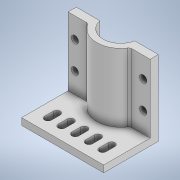
# Autodesk Inventor part: CLAMP
Saved by Autodesk Inventor 2022 (Build 260153000, 153)
## iProperties
Created: 2022-02-10
Part Number: CLAMP
Material: Generic
Document SubType Name: Modeling
Designer: 24sa01
Density: 1 g/cm^3
Appearance: Default
Author: 24sa01
Autodesk Inventor part; units mm, degrees
ref_plane "YZ Plane" through (0, 0, 0) normal (1, 0, 0) x (0, 1, 0)
ref_plane "XZ Plane" through (0, 0, 0) normal (0, 1, 0) x (-1, 0, 0)
ref_plane "XY Plane" through (0, 0, 0) normal (0, 0, 1) x (1, 0, 0)
sketch "Sketch1" plane through (0, 0, 0) normal (0, 1, 0) x (-1, 0, 0)
  line L0 (0, 0) -> (-76.2, 0)
  line L1 (-76.2, 0) -> (-76.2, -50.8)
  line L2 (-76.2, -50.8) -> (0, -50.8)
  line L3 (0, -50.8) -> (0, 0)
  line L4 (-12.7, -11.7475) -> (-12.7, -20.0025) construction
  line L5 (-15.875, -11.7475) -> (-15.875, -20.0025)
  line L6 (-9.525, -20.0025) -> (-9.525, -11.7475)
  arc A0 (-9.525, -11.7475) -> (-15.875, -11.7475) centre (-12.7, -11.7475) ccw
  arc A1 (-15.875, -20.0025) -> (-9.525, -20.0025) centre (-12.7, -20.0025) ccw
  line L7 (-25.4, -11.7475) -> (-25.4, -20.0025) construction
  line L8 (-28.575, -11.7475) -> (-28.575, -20.0025)
  line L9 (-22.225, -20.0025) -> (-22.225, -11.7475)
  arc A2 (-22.225, -11.7475) -> (-28.575, -11.7475) centre (-25.4, -11.7475) ccw
  arc A3 (-28.575, -20.0025) -> (-22.225, -20.0025) centre (-25.4, -20.0025) ccw
  line L10 (-28.575, -11.7475) -> (-28.575, -20.0025)
  line L11 (-25.4, -11.7475) -> (-25.4, -20.0025) construction
  arc A4 (-22.225, -11.7475) -> (-28.575, -11.7475) centre (-25.4, -11.7475) ccw
  line L12 (-22.225, -20.0025) -> (-22.225, -11.7475)
  arc A5 (-28.575, -20.0025) -> (-22.225, -20.0025) centre (-25.4, -20.0025) ccw
  line L13 (-41.275, -11.7475) -> (-41.275, -20.0025)
  line L14 (-38.1, -11.7475) -> (-38.1, -20.0025) construction
  arc A6 (-34.925, -11.7475) -> (-41.275, -11.7475) centre (-38.1, -11.7475) ccw
  line L15 (-34.925, -20.0025) -> (-34.925, -11.7475)
  arc A7 (-41.275, -20.0025) -> (-34.925, -20.0025) centre (-38.1, -20.0025) ccw
  line L16 (-53.975, -11.7475) -> (-53.975, -20.0025)
  line L17 (-50.8, -11.7475) -> (-50.8, -20.0025) construction
  arc A8 (-47.625, -11.7475) -> (-53.975, -11.7475) centre (-50.8, -11.7475) ccw
  line L18 (-47.625, -20.0025) -> (-47.625, -11.7475)
  arc A9 (-53.975, -20.0025) -> (-47.625, -20.0025) centre (-50.8, -20.0025) ccw
  line L19 (-66.675, -11.7475) -> (-66.675, -20.0025)
  line L20 (-63.5, -11.7475) -> (-63.5, -20.0025) construction
  arc A10 (-60.325, -11.7475) -> (-66.675, -11.7475) centre (-63.5, -11.7475) ccw
  line L21 (-60.325, -20.0025) -> (-60.325, -11.7475)
  arc A11 (-66.675, -20.0025) -> (-60.325, -20.0025) centre (-63.5, -20.0025) ccw
  point P0 (-12.7, -15.875)
  point P1 (-25.4, -15.875)
  point P2 (-25.4, -15.875)
  point P3 (-38.1, -15.875)
  point P4 (-50.8, -15.875)
  point P5 (-63.5, -15.875)
  dimension "d0" = 50.8
  dimension "d1" = 76.2
  dimension "d41" = 8.255
  dimension "d42" = 6.35
  dimension "d43" = 12.7
  dimension "d44" = 8.255
  dimension "d45" = 6.35
  dimension "d56" = 12.7
  dimension "d57" = 15.875
  dimension "d60" = 12.7
  constraints: 56 end point, 24 point on circle, 12 centre point, 8 tangent, 4 parallel, 2 horizontal, 2 midpoint, 2 vertical, 1 horizontal alignment, 1 perpendicular, 48 other
  measures "d0" distance of L0.end L1.end
  measures "d1" distance of L1.end L2.end
  measures "d41" distance of L4.start L4.end
  measures "d42" diameter of A1
  measures "d43" distance from line of L3 point (-12.7, -15.875)
  measures "d44" distance of L7.start L7.end
  measures "d45" diameter of A3
  measures "d56" distance of point (-25.4, -15.875) point (-12.7, -15.875)
  measures "d57" distance from line of point (-12.7, -15.875) L0
  measures "d60" distance of L5.start L10.start
extrude "Extrusion1" add sketch "Sketch1" along normal blind 6.35
sketch "Sketch2" plane through (0, 6.35, 0) normal (0, 1, 0) x (1, 0, 0)
  line L0 (76.2, 50.8) -> (0, 50.8)
  circle A0 centre (38.1, 53.975) radius 16.51
  line L1 (0, 50.8) -> (0, 0) projected
  circle A1 centre (38.1, 53.975) radius 22.225
  line L2 (18.6727, 43.18) -> (0, 43.18)
  line L3 (76.2, 50.8) -> (0, 50.8) projected
  line L4 (57.5273, 43.18) -> (76.2, 43.18)
  line L5 (76.2, 0) -> (76.2, 50.8) projected
  point P0 (54.3018, 50.8)
  point P1 (21.8982, 50.8)
  dimension "d22" = 33.02
  dimension "d23" = 3.175
  dimension "d24" = 38.1
  dimension "d25" = 44.45
  dimension "d26" = 7.62
  dimension "d27" = 7.62
  constraints: 6 end point, 2 centre point, 2 point on circle, 2 point on line, 1 coincident, 1 horizontal, 1 perpendicular
  measures "d22" diameter of A0
  measures "d23" distance from line of L0 A0.centre
  measures "d24" distance from line of L1 A0.centre
  measures "d25" diameter of A1
  measures "d26" distance between parallel lines of L0 L2
  measures "d27" distance between parallel lines of L0 L4
extrude "Extrusion2" add sketch "Sketch2" along normal blind 63.5 contours L5 L4 A1 L0 | A1 L0 A0 | L2 L1 L0 A1 picked at (21.7987, 42.02)
sketch "Sketch3" plane through (0, 6.35, -43.18) normal (0, 0, 1) x (1, 0, 0)
  line L0 (76.2, 0) -> (76.2, 63.5) projected
  line L1 (0, 0) -> (0, 63.5) projected
  line L2 (0, 63.5) -> (18.6727, 63.5) projected
  line L3 (57.5273, 63.5) -> (76.2, 63.5) projected
  line L4 (54.3018, 0) -> (21.8982, 0) projected
  point P0 (0, -6.35)
  point P1 (6.35, 44.45)
  point P2 (69.85, 44.45)
  point P3 (6.35, 19.05)
  point P4 (69.85, 19.05)
  dimension "d30" = 6.35
  dimension "d31" = 6.35
  dimension "d32" = 19.05
  dimension "d33" = 19.05
  dimension "d52" = 6.35
  dimension "d53" = 6.35
  dimension "d54" = 19.05
  dimension "d55" = 19.05
  measures "d30" distance from line of L0 point (69.85, 44.45)
  measures "d31" distance from line of L1 point (6.35, 44.45)
  measures "d32" distance from line of L2 point (6.35, 44.45)
  measures "d33" distance from line of L3 point (69.85, 44.45)
  measures "d52" distance from line of L1 point (6.35, 19.05)
  measures "d53" distance from line of L0 point (69.85, 19.05)
  measures "d54" distance from line of L4 point (69.85, 19.05)
  measures "d55" distance from line of L4 point (6.35, 19.05)
hole "Hole1" at (6.35, 50.8, -43.18) at (6.35, 25.4, -43.18) at (69.85, 25.4, -43.18) at (69.85, 50.8, -43.18) direction (0, 0, -1) diameter 6.7564 end through all
fillet "Fillet1" radius 3.175 2 edges at (18.6727, 38.1, -43.18) (57.5273, 38.1, -43.18)
sketch "Sketch6" plane through (0, 6.35, 0) normal (0, 1, 0) x (1, 0, 0)
  circle A0 centre (38.1, 53.975) radius 16.51
  arc A1 (21.8982, 50.8) -> (54.3018, 50.8) centre (38.1, 53.975) ccw projected
  point P0 (0, 0)
  dimension "d49" = 33.02
  constraints: 1 centre point, 1 concentric
  measures "d49" diameter of A0
extrude "Extrusion3" cut sketch "Sketch6" against normal blind 25.4
body "Solid1"
